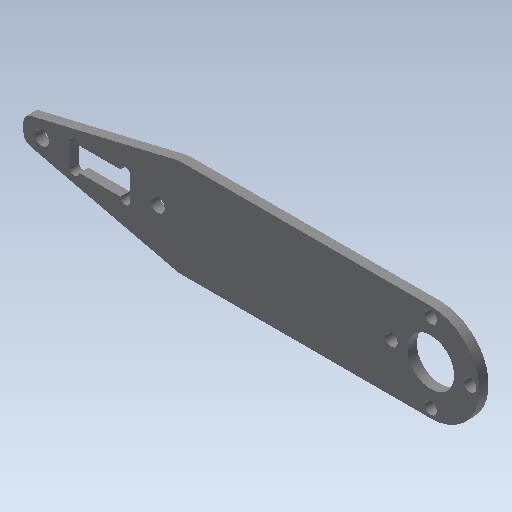
# Autodesk Inventor part: 前腕_メインフレーム_1_2
Saved by Autodesk Inventor 2020.3 (Build 243373000, 373)
## iProperties
Created: 2016-05-04
Part Number: 前腕_メインフレーム_1_2
Material: GFRP
Document SubType Name: Modeling
Designer: hiroaki
Density: 1.75 g/cm^3
Appearance: 滑らか - 淡い灰色
Mass: 5.45877 g
Surface Area: 38.0175 cm^2
Volume: 3.11929 cm^3
Category: 前腕
d0: 200.000 mm
d1: 3.100 mm
d2: 21.000 mm
d3: 10.000 mm
d4: 5.000 mm
d5: 12.000 mm
d6: 135.000 mm
d7: 5.000 mm
d8: 0.050 mm
d9: 2.100 mm
d10: 2.700 mm
d11: 8.500 mm
d12: 10.100 mm
d13: 4.000 ul
d15: 360.00 deg
d17: 2.000 mm
d18: 0.00 deg
Author: hiroaki
Autodesk Inventor part; units mm, degrees
ref_plane "YZ Plane" through (0, 0, 0) normal (1, 0, 0) x (0, 1, 0)
ref_plane "XZ Plane" through (0, 0, 0) normal (0, 1, 0) x (-1, 0, 0)
ref_plane "XY Plane" through (0, 0, 0) normal (0, 0, 1) x (1, 0, 0)
sketch "スケッチ1" plane through (0, 0, 0) normal (0, 0, 1) x (1, 0, 0)
  circle A0 centre (0, 0) radius 10.5 construction
  line L0 (0, 10.5) -> (-200, 10.5) construction
  line L1 (-200, 10.5) -> (-200, -10.5) construction
  line L2 (-200, -10.5) -> (0, -10.5) construction
  circle A1 centre (-195, 0) radius 1.55 construction
  line L3 (-185, 2.5) -> (-70, 2.5) construction
  line L4 (-70, 2.5) -> (-70, -2.5) construction
  line L5 (-70, -2.5) -> (-185, -2.5) construction
  line L6 (-185, -2.5) -> (-185, 2.5) construction
  line L7 (-127.5, 2.5) -> (-127.5, -2.5) construction
  circle A2 centre (-60, 0) radius 1.55 construction
  line L8 (-12, 21.3027) -> (-12, -27.3903) construction
  line L9 (-69.95, 2.55) -> (-185.05, 2.55) construction
  line L10 (-185.05, 2.55) -> (-185.05, -2.55) construction
  line L11 (-185.05, -2.55) -> (-69.95, -2.55) construction
  line L12 (-69.95, -2.55) -> (-69.95, 2.55) construction
  circle A3 centre (-184, 2.55) radius 1.05 construction
  line L13 (-185, 0) -> (-127.5, 0) construction
  line L14 (-185.05, 2.55) -> (-185.05, -2.55) construction
  arc A4 (-182.95, 2.55) -> (-185.05, 2.55) centre (-184, 2.55) ccw construction
  line L15 (-182.95, 2.55) -> (-72.05, 2.55) construction
  arc A5 (-69.95, 2.55) -> (-72.05, 2.55) centre (-71, 2.55) ccw construction
  line L16 (-69.95, 2.55) -> (-69.95, -2.55) construction
  arc A6 (-185.05, -2.55) -> (-182.95, -2.55) centre (-184, -2.55) ccw construction
  line L17 (-182.95, -2.55) -> (-72.05, -2.55) construction
  arc A7 (-72.05, -2.55) -> (-69.95, -2.55) centre (-71, -2.55) ccw construction
  circle A8 centre (0, 8.5) radius 1.35
  circle A9 centre (0, 0) radius 5.05
  circle A10 centre (-8.5, 0) radius 1.35
  circle A11 centre (0, -8.5) radius 1.35
  circle A12 centre (8.5, 0) radius 1.35
  line L18 (-200, 4.8006) -> (-200, -4.8006) construction
  line L19 (-200, 4.8006) -> (-60, 10.5) construction
  line L20 (-60, 10.5) -> (0, 10.5) construction
  line L21 (-200, -4.8006) -> (-60, -10.5) construction
  line L22 (-60, -10.5) -> (0, -10.5) construction
  arc A13 (0, -10.5) -> (0, 10.5) centre (0, 0) ccw construction
  circle A14 centre (-195, 0) radius 5 construction
  circle A15 centre (-59, 0) radius 1.55
  circle A16 centre (-84, 0) radius 1.55
  line L23 (-55, -2.5) -> (-88, -2.5) construction
  line L24 (-88, -2.5) -> (-88, 2.5) construction
  line L25 (-88, 2.5) -> (-55, 2.5) construction
  line L26 (-55, 2.5) -> (-55, -2.5) construction
  line L27 (-65, -2.5) -> (-78, -2.5) construction
  line L28 (-78, -2.5) -> (-78, 2.5) construction
  line L29 (-78, 2.5) -> (-65, 2.5) construction
  line L30 (-65, 2.5) -> (-65, -2.5) construction
  line L31 (-64.95, -2.55) -> (-78.05, -2.55)
  line L32 (-78.05, -2.55) -> (-78.05, 2.55)
  line L33 (-78.05, 2.55) -> (-64.95, 2.55)
  line L34 (-64.95, 2.55) -> (-64.95, -2.55)
  circle A17 centre (-66, -2.55) radius 1.05
  circle A18 centre (-66, 2.55) radius 1.05
  circle A19 centre (-77, -2.55) radius 1.05
  circle A20 centre (-77, 2.55) radius 1.05
  line L35 (-88, 2.5) -> (-88, -2.5)
  line L36 (-88, -2.5) -> (-54.4113, -10.5)
  line L37 (-88, 2.5) -> (-54.4113, 10.5)
  arc A21 (0, -10.5) -> (0, 10.5) centre (0, 0) ccw
  line L38 (-54.4113, 10.5) -> (0, 10.5)
  line L39 (0, -10.5) -> (-54.4113, -10.5)
  circle A22 centre (-77, 2.55) radius 2.5 construction
  circle A23 centre (0, 0) radius 16 construction
  circle A24 centre (0, 0) radius 21 construction
  line L40 (-21, 19.3585) -> (-21, -28.09) construction
  point P0 (-200, 0)
  point P1 (-55, 0)
  dimension "d9" = 2.1
  dimension "d29" = 2.1
  dimension "d0" = 200
  dimension "d1" = 3.1
  dimension "d2" = 21
  dimension "d3" = 10
  dimension "d4" = 5
  dimension "d5" = 12
  dimension "d6" = 135
  dimension "d7" = 5
  dimension "d8" = 0.05
  dimension "d10" = 2.7
  dimension "d11" = 8.5
  dimension "d12" = 10.1
  dimension "d15" = 360
  dimension "d20" = 3.1
  dimension "d21" = 5
  dimension "d22" = 4
  dimension "d23" = 5
  dimension "d24" = 25
  dimension "d26" = 10
  dimension "d27" = 4
  dimension "d28" = 10
  dimension "d30" = 0.05
  dimension "d32" = 5
  dimension "d33" = 32
  dimension "d34" = 5
  constraints: 82 end point, 19 centre point, 14 point on circle, 11 horizontal alignment, 11 tangent, 10 parallel, 9 coincident, 9 horizontal, 8 perpendicular, 7 midpoint, 5 collinear, 5 point on line, 5 symmetric about line, 5 vertical, 4 equal radius, 3 vertical alignment, 2 concentric, 30 other
  measures "d0" distance from line of L1 point (0, 0)
  measures "d1" diameter of A1
  measures "d2" distance of L0.end L1.end
  measures "d3" distance from line of L6 A1.centre
  measures "d4" distance from line of L1 A1.centre
  measures "d5" distance from line of point (0, 0) L8
  measures "d6" distance of A2.centre A1.centre
  measures "d7" distance of L3.end L4.end
  measures "d8" distance between parallel lines of L9 L3
  measures "d10" diameter of A8
  measures "d11" distance of point (0, 0) A8.centre
  measures "d12" diameter of A9
  measures "d20" diameter of A15
  measures "d21" distance from line of L26 A2.centre
  measures "d22" distance from line of L26 A15.centre
  measures "d23" distance of L25.end L23.start
  measures "d24" distance of A16.centre A15.centre
  measures "d26" distance between parallel lines of L30 L26
  measures "d27" distance from line of A16.centre L24
  measures "d28" distance between parallel lines of L28 L24
  measures "d30" distance between parallel lines of L34 L30
  measures "d32" diameter of A22
  measures "d33" diameter of A23
  measures "d34" radial gap between concentric circles of A24 A23
extrude "押し出し1" add sketch "スケッチ1" along normal blind 2
fillet "フィレット2" radius 2 2 edges at (-88, 2.5, 1) (-88, -2.5, 1)
equation "\"d0\" = d0_1"
equation "\"d2\" = d2_1"
equation "\"d3\" = d3_1"
equation "\"d4\" = d4_1"
equation "\"d6\" = d6_1"
equation "\"d21\" = d4"
equation "\"d27\" = d22"
equation "\"d28\" = d26"
equation "\"d2_1\" = 21"
equation "\"d3_1\" = 10"
equation "\"d4_1\" = 5"
equation "\"d6_1\" = 135"
equation "\"d0_1\" = 200"
